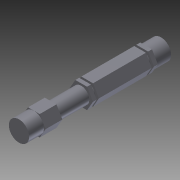
# Autodesk Inventor part: shaft - step down No. 2
Saved by Autodesk Inventor 2012 (Build 160160000, 160)
## iProperties
Created: 2012-02-05
Part Number: shaft - step down No. 2
Material: Steel
Document SubType Name: Modeling
Designer: Antonella Wilby
Mass: 55.7021 g
Surface Area: 25.1426 cm^2
Volume: 7.09581 cm^3
Density: 7.85 g/cm^3
Author: Antonella Wilby
Autodesk Inventor part; units mm, degrees
ref_plane "YZ Plane" through (0, 0, 0) normal (1, 0, 0) x (0, 1, 0)
ref_plane "XZ Plane" through (0, 0, 0) normal (0, 1, 0) x (-1, 0, 0)
ref_plane "XY Plane" through (0, 0, 0) normal (0, 0, 1) x (1, 0, 0)
sketch "Sketch1" plane through (0, 0, 0) normal (0, 0, 1) x (1, 0, 0)
  line L0 (-7.699, 0) -> (7.699, 0) projected
  line L1 (0, -6.6675) -> (0, 6.6675) projected
  line L2 (2.7496, 4.7625) -> (5.4993, 0)
  line L3 (5.4993, 0) -> (2.7496, -4.7625)
  line L4 (2.7496, -4.7625) -> (-2.7496, -4.7625)
  line L5 (-2.7496, -4.7625) -> (-5.4993, 0)
  line L6 (-5.4993, 0) -> (-2.7496, 4.7625)
  line L7 (-2.7496, 4.7625) -> (2.7496, 4.7625)
  point P0 (0, 0)
  point P1 (0, 0)
  point P2 (0, 4.7625)
  dimension "d0" = 9.525
  constraints: 12 end point, 1 coincident, 1 midpoint, 1 vertical alignment, 13 other
  measures "d0" distance between parallel lines of L7 L4
extrude "Extrusion1" add sketch "Sketch1" along normal mid plane 66.675
sketch "Sketch2" plane through (0, 0, 33.3375) normal (0, 0, 1) x (1, 0, 0)
  line L0 (5.4993, 0) -> (2.7496, -4.7625) projected
  line L1 (2.7496, 4.7625) -> (5.4993, 0) projected
  line L2 (-2.7496, 4.7625) -> (2.7496, 4.7625) projected
  line L3 (-5.4993, 0) -> (-2.7496, 4.7625) projected
  line L4 (-2.7496, -4.7625) -> (-5.4993, 0) projected
  line L5 (2.7496, -4.7625) -> (-2.7496, -4.7625) projected
  circle A0 centre (0, 0) radius 4.7625
  constraints: 1 centre point, 1 coincident, 1 tangent
extrude "Extrusion2" cut sketch "Sketch2" against normal blind 6.985 contours L0 A0 L1 | L0 L5 A0 | A0 L2 L1 | L5 L4 A0 | A0 L3 L2 | L4 L3 A0
mirror "Mirror1" about plane through (0, 0, 0) normal (0, 0, 1) of "Extrusion2"
ref_plane "Work Plane2" through (0, 0, -23.5077) normal (0, 0, -1) x (-1, 0, 0)
sketch "Sketch3" plane through (0, 0, -23.5077) normal (0, 0, -1) x (-1, 0, 0)
  circle A0 centre (0, 0) radius 3.8481
  line L0 (-2.7496, 4.7625) -> (0, 4.7625) projected
  line L1 (-4.1244, 2.3813) -> (-2.7496, 4.7625) projected
  circle A1 centre (0, 0) radius 5.4993
  dimension "d7" = 7.6962
  constraints: 2 coincident, 1 centre point, 3 other
  measures "d7" diameter of A0
extrude "Extrusion3" cut sketch "Sketch3" along normal blind 0.9906
ref_plane "Work Plane3" through (0, 0, 1.3335) normal (0, 0, -1) x (-1, 0, 0)
sketch "Sketch4" plane through (0, 0, 1.3335) normal (0, 0, -1) x (-1, 0, 0)
  line L0 (-2.7496, 4.7625) -> (0, 4.7625) projected
  line L1 (-4.1244, 2.3813) -> (-2.7496, 4.7625) projected
  circle A0 centre (0, 0) radius 3.8481
  circle A1 centre (0, 0) radius 5.4993
  dimension "d12" = 7.6962
  constraints: 2 coincident, 1 centre point, 3 other
  measures "d12" diameter of A0
extrude "Extrusion4" cut sketch "Sketch4" against normal blind 0.9906
ref_plane "Work Plane5" through (0, 0, 18.4785) normal (0, 0, 1) x (1, 0, 0)
sketch "Sketch5" plane through (0, 0, 18.4785) normal (0, 0, 1) x (1, 0, 0)
  line L0 (-2.7496, 4.7625) -> (0, 4.7625) projected
  line L1 (-4.1244, 2.3813) -> (-2.7496, 4.7625) projected
  circle A0 centre (0, 0) radius 5.4993
  circle A1 centre (0, 0) radius 3.81
  dimension "d17" = 7.62
  constraints: 2 coincident, 1 centre point, 3 other
  measures "d17" diameter of A1
extrude "Extrusion5" cut sketch "Sketch5" against normal blind 14.351
body "Solid1"
